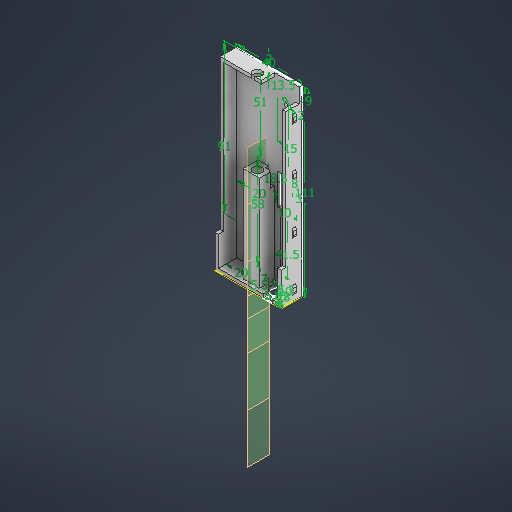
# Autodesk Inventor part: editable_tray
Saved by Autodesk Inventor 2026.2 (Build 302298000, 298)
## iProperties
Created: 2025-11-10
Part Number: editable_tray
Material: Generic
Document SubType Name: Modeling
Designer: SCANTURK
Density: 1 g/cm^3
Appearance: Default
Author: SCANTURK
Autodesk Inventor part; units mm, degrees
ref_plane "YZ Plane" through (0, 0, 0) normal (1, 0, 0) x (0, 1, 0)
ref_plane "XZ Plane" through (0, 0, 0) normal (0, 1, 0) x (-1, 0, 0)
ref_plane "XY Plane" through (0, 0, 0) normal (0, 0, 1) x (1, 0, 0)
sketch "Sketch1" plane through (0, 0, 0) normal (0, 0, 1) x (1, 0, 0)
  line L0 (0, 0) -> (40, 0)
  line L1 (40, 0) -> (40, 111)
  line L2 (40, 111) -> (0, 111)
  line L3 (0, 111) -> (0, 0)
  line L4 (2, 109) -> (38, 109)
  line L5 (38, 109) -> (38, 2)
  line L6 (38, 2) -> (2, 2)
  line L7 (2, 2) -> (2, 109)
  line L8 (25, 111) -> (25, 109)
  line L9 (38, 102) -> (40, 102)
  line L10 (0, 20) -> (2, 20)
  line L11 (38, 20) -> (40, 20)
  circle A0 centre (32, 97.5) radius 1
  line L12 (27, 60) -> (37, 60)
  line L13 (37, 60) -> (37, 41.5)
  line L14 (37, 41.5) -> (27, 41.5)
  line L15 (27, 41.5) -> (27, 60)
  line L16 (15, 60) -> (25, 60)
  line L17 (25, 60) -> (25, 2)
  line L18 (25, 2) -> (15, 2)
  line L19 (15, 2) -> (15, 60)
  line L20 (25, 60) -> (21.338, 60)
  line L21 (25, 51.5) -> (25, 60)
  point P0 (25, 110)
  point P1 (39, 102)
  point P2 (1, 20)
  point P3 (32, 41.5)
  point P4 (20, 60)
  dimension "d0" = 40
  dimension "d1" = 111
  dimension "d2" = 2
  dimension "d3" = 15
  dimension "d4" = 9
  dimension "d5" = 91
  dimension "d6" = 2
  dimension "d7" = 13.5
  dimension "d8" = 8
  dimension "d9" = 10
  dimension "d10" = 18.5
  dimension "d11" = 3
  dimension "d12" = 41.5
  dimension "d13" = 10
  dimension "d14" = 58
  dimension "d17" = 20
  dimension "d80" = 51
  constraints: 44 end point, 10 point on line, 8 parallel, 7 perpendicular, 5 midpoint, 4 horizontal, 1 centre point, 3 other
  measures "d0" distance of L2.end L1.end
  measures "d1" distance of L1.end L0.end
  measures "d2" distance between parallel lines of L2 L4
  measures "d3" distance from line of L1 point (25, 110)
  measures "d4" distance from line of point (39, 102) L2
  measures "d5" distance from line of point (1, 20) L2
  measures "d6" diameter of A0
  measures "d7" distance from line of L2 A0.centre
  measures "d8" distance from line of L1 A0.centre
  measures "d9" distance of L13.end L14.end
  measures "d10" distance of L14.end L12.start
  measures "d11" distance between parallel lines of L13 L1
  measures "d12" distance from line of L0 point (32, 41.5)
  measures "d13" distance of L17.end L18.end
  measures "d14" distance of L18.end L16.start
  measures "d17" distance from line of L3 point (20, 60)
  measures "d80" distance between parallel lines of L2 L16
extrude "Extrusion1" add sketch "Sketch1" along normal blind 1.6
extrude "Extrusion3" add sketch "Sketch1" along normal blind 8 from surface at 1.6 contours L3 L10 L7 L6 L5 L11 L1 L0 | L3 L2 L8 L4 L7 L10 | L11 L5 L9 L1
extrude "Extrusion4" add sketch "Sketch1" along normal blind 3 from surface at 9.6 contours L3 L10 L7 L6 L5 L11 L1 L0
extrude "Extrusion5" add sketch "Sketch1" along normal blind 9 from surface at 1.6 contours L19 L16 L17 L6
sketch "Sketch3" plane through (0, 0, 0) normal (0, -1, 0) x (1, 0, 0)
  circle A0 centre (20, 7) radius 2.75
  circle A1 centre (32, 5.5) radius 5
  line L0 (0, 0) -> (0, 12.6) projected
  line L1 (0, 0) -> (40, 0) projected
  line L2 (40, 0) -> (40, 12.6) projected
  line L3 (40, 12.6) -> (0, 12.6) projected
  line L4 (29.095, 12.6) -> (34.905, 12.6)
  line L5 (34.905, 12.6) -> (34.905, 8.6)
  line L6 (34.905, 8.6) -> (29.095, 8.6)
  line L7 (29.095, 8.6) -> (29.095, 12.6)
  point P0 (32, 8.6)
  point P1 (29.095, 9.5695)
  point P2 (34.905, 9.5695)
  dimension "d49" = 5.5
  dimension "d50" = 10
  dimension "d51" = 20
  dimension "d52" = 7
  dimension "d53" = 8
  dimension "d54" = 5.5
  dimension "d81" = 5.81
  dimension "d82" = 4
  dimension "d83" = 8
  constraints: 8 end point, 2 centre point, 2 parallel, 1 horizontal, 1 midpoint, 1 perpendicular, 1 point on line
  measures "d49" diameter of A0
  measures "d50" diameter of A1
  measures "d51" distance from line of L0 A0.centre
  measures "d52" distance from line of L1 A0.centre
  measures "d53" distance from line of A1.centre L2
  measures "d54" distance from line of L1 A1.centre
  measures "d81" distance of L5.end L6.end
  measures "d82" distance of L4.end L5.end
  measures "d83" distance from line of L2 point (32, 8.6)
extrude "Extrusion6" cut sketch "Sketch3" against normal up to surface (111 mm away) from surface at 0 contours A0
sketch "Sketch4" plane through (15, 60, 1.6) normal (0, 1, 0) x (1, 0, 0)
  line L0 (0, 0) -> (10, 0) projected
  line L1 (10, 0) -> (6.338, 0)
  line L2 (6.338, 0) -> (6.338, -1.771)
  line L3 (6.338, -1.771) -> (10, -1.771)
  line L4 (10, -1.771) -> (10, 0)
  line L5 (10, 0) -> (10, -2.6)
  line L6 (10, 0) -> (10, -9) projected
  line L7 (6.338, -1.771) -> (8.214, -1.771)
  line L8 (8.214, -1.771) -> (10, -2.6)
  point P0 (-15, 1.6)
  point P1 (6.338, 0)
  point P2 (10, -11)
  dimension "d57" = 1.771
  dimension "d58" = 3.662
  dimension "d59" = 2.6
  dimension "d60" = 1.876
  constraints: 14 end point, 2 parallel, 2 point on line, 1 horizontal, 1 perpendicular
  measures "d57" distance of L1.end L2.end
  measures "d58" distance of L2.end L3.end
  measures "d59" distance of L0.end L5.end
  measures "d60" distance of L2.end L7.end
extrude "Extrusion7" cut sketch "Sketch4" against normal blind 8.5
extrude "Extrusion8" cut sketch "Sketch3" against normal up to surface (41.5 mm away) contours A1 L7 L6 L5 | L5 L6 L7 A1 | A1 L7 L3 L5
sketch "Sketch5" plane through (0, 0, 0) normal (1, 0, 0) x (0, 0, -1)
  line L0 (-5.8, 93.5) -> (-3.8, 93.5)
  line L1 (-3.8, 93.5) -> (-3.8, 98.5)
  line L2 (-3.8, 98.5) -> (-5.8, 98.5)
  line L3 (-5.8, 98.5) -> (-5.8, 93.5)
  line L4 (-5.8, 93.5) -> (-3.8, 98.5) construction
  line L5 (-3.8, 93.5) -> (-5.8, 98.5) construction
  line L6 (0, 111) -> (-1.6, 111) projected
  line L7 (0, 0) -> (0, 111) projected
  point P0 (-4.8, 96)
  dimension "d65" = 2
  dimension "d66" = 5
  dimension "d67" = 15
  dimension "d68" = 4.8
  constraints: 12 end point, 2 midpoint, 2 parallel, 1 horizontal, 1 perpendicular
  measures "d65" distance of L2.end L1.end
  measures "d66" distance of L1.end L0.end
  measures "d67" distance from line of L6 point (-4.8, 96)
  measures "d68" distance from line of L7 point (-4.8, 96)
extrude "Extrusion9" add sketch "Sketch5" against normal blind 0.5
sketch "Sketch6" plane through (0, 93.5, 5.8) normal (0, 0, 1) x (1, 0, 0)
  line L0 (-0.5, 5) -> (-0.5, 0) projected
  line L1 (-0.5, 5) -> (0, 5)
  line L2 (0, 5) -> (0, 0)
  line L3 (0, 0) -> (-0.5, 0)
  line L4 (-0.5, 0) -> (-0.5, 5)
  line L5 (0, 0) -> (-0.5, 0.2887)
  line L6 (0, 5) -> (-0.5, 4.7113)
  point P0 (0, -93.5)
  point P1 (-0.5, 0.2887)
  point P2 (-0.5, 4.7113)
  dimension "d72" = 60
  dimension "d73" = 60
  constraints: 12 end point, 2 parallel, 2 point on line, 1 horizontal, 1 perpendicular
  measures "d72" angle of L2 L5
  measures "d73" angle of L2 L6
extrude "Extrusion10" cut sketch "Sketch6" against normal up to surface (2 mm away) contours L1 L6 L0 | L5 L3 L0
fillet "Fillet1" radius 2 2 edges at (-0.5, 93.7887, 4.8) (-0.5, 98.2113, 4.8)
ref_plane "Work Plane1" through (20, 0, 0) normal (-1, 0, 0) x (0, 0, 1)
mirror "Mirror1" about plane through (20, 0, 0) normal (-1, 0, 0) of "Extrusion9", "Extrusion10", "Fillet1"
pattern_linear "Rectangular Pattern1" count 4 spacing -30 along (0, 1, 0) of "Extrusion9", "Extrusion10", "Fillet1", "Mirror1"
ref_plane "Work Plane2" through (20, 0, 0) normal (-1, 0, 0) x (0, 0, 1)
ref_plane "Work Plane3" through (20, -30, 0) normal (-1, 0, 0) x (0, 0, 1)
ref_plane "Work Plane4" through (20, -30, 0) normal (-1, 0, 0) x (0, 0, 1)
ref_plane "Work Plane5" through (20, -60, 0) normal (-1, 0, 0) x (0, 0, 1)
ref_plane "Work Plane6" through (20, -90, 0) normal (-1, 0, 0) x (0, 0, 1)
ref_plane "Work Plane7" through (20, -60, 0) normal (-1, 0, 0) x (0, 0, 1)
ref_plane "Work Plane8" through (20, -90, 0) normal (-1, 0, 0) x (0, 0, 1)
body "Solid1"
